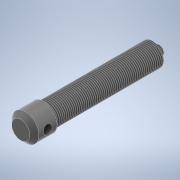
# Autodesk Inventor part: Prisioneiro
Saved by Autodesk Inventor 2021 (Build 250183000, 183)
## iProperties
Created: 2021-05-13
Part Number: Prisioneiro
Material: Genérico
Document SubType Name: Modeling
Designer: rubia
Density: 1 g/cm^3
Appearance: Liso - Preto
Author: rubia
Autodesk Inventor part; units mm, degrees
ref_plane "YZ Plane" through (0, 0, 0) normal (1, 0, 0) x (0, 1, 0)
ref_plane "XZ Plane" through (0, 0, 0) normal (0, 1, 0) x (-1, 0, 0)
ref_plane "XY Plane" through (0, 0, 0) normal (0, 0, 1) x (1, 0, 0)
sketch "Esboço1" plane through (0, 0, 0) normal (0, 0, 1) x (1, 0, 0)
  circle A0 centre (0, 0) radius 25
  dimension "d0" = 50
  constraints: 1 centre point, 1 coincident
  measures "d0" diameter of A0
extrude "Extrusão1" add sketch "Esboço1" along normal blind 240
sketch "Esboço2" plane through (0, 0, 240) normal (0, 0, 1) x (1, 0, 0)
  circle A0 centre (0, 0) radius 30
  dimension "d3" = 60
  constraints: 1 centre point, 1 coincident
  measures "d3" diameter of A0
extrude "Extrusão2" add sketch "Esboço2" along normal blind 50
chamfer "Chanfro1" distance 10 angle 45 1 edges at (-30, 0, 290)
thread "Rosca1" size "M50x4" class "6g" standard "ANSI Metric M Profile" length 240
sketch "Esboço3" plane through (0, 0, 0) normal (1, 0, 0) x (0, 1, 0)
  line L0 (30, 280) -> (-30, 280) construction
  line L1 (30, 240) -> (-30, 240) construction
  line L2 (30, 280) -> (-30, 240) construction
  line L3 (30, 240) -> (-30, 280) construction
  circle A0 centre (0, 260) radius 10
  point P0 (0, 0)
  dimension "d11" = 20
  constraints: 4 end point, 1 centre point, 1 midpoint
  measures "d11" diameter of A0
extrude "Extrusão3" cut sketch "Esboço3" along normal through all both and the other way through all
sketch "Esboço4" plane through (0, 0, 0) normal (0, 0, -1) x (-1, 0, 0)
  circle A0 centre (0, 0) radius 10
  dimension "d14" = 20
  constraints: 1 centre point, 1 coincident
  measures "d14" diameter of A0
extrude "Extrusão4" add sketch "Esboço4" along normal blind 15
